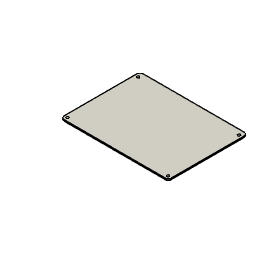
Under Table Mainboard Case - Lid (Autodesk Fusion 360 design; units mm, degrees)
Autodesk Fusion 360 part; units mm, degrees
sketch "Sketch1" plane through (0, 0, 63) normal (0, 0, 1) x (-1, 0, 0)
  circle A0 centre (89, -61) radius 1.925
  circle A1 centre (89, 64) radius 1.925
  circle A2 centre (-89, -61) radius 1.925
  circle A3 centre (-89, 64) radius 1.925
  line L0 (-89, -68.4) -> (-85, -68.4)
  line L1 (-85, -68.4) -> (-85, -67)
  line L2 (-85, -67) -> (-74, -67)
  line L3 (-74, -67) -> (-74, -64)
  line L4 (-74, -64) -> (-83, -64)
  arc A4 (-86, -61) -> (-83, -64) centre (-83, -61) ccw
  arc A5 (-86, -61) -> (-89, -58) centre (-89, -61) ccw
  arc A6 (-92, -55) -> (-89, -58) centre (-89, -55) ccw
  line L5 (-92, -55) -> (-92, 58)
  arc A7 (-89, 61) -> (-92, 58) centre (-89, 58) ccw
  arc A8 (-89, 61) -> (-86, 64) centre (-89, 64) ccw
  arc A9 (-83, 67) -> (-86, 64) centre (-83, 64) ccw
  line L6 (-83, 67) -> (83, 67)
  arc A10 (86, 64) -> (83, 67) centre (83, 64) ccw
  arc A11 (86, 64) -> (89, 61) centre (89, 64) ccw
  arc A12 (92, 58) -> (89, 61) centre (89, 58) ccw
  line L7 (92, 58) -> (92, -55)
  arc A13 (89, -58) -> (92, -55) centre (89, -55) ccw
  arc A14 (89, -58) -> (86, -61) centre (89, -61) ccw
  arc A15 (83, -64) -> (86, -61) centre (83, -61) ccw
  line L8 (83, -64) -> (74, -64)
  line L9 (74, -64) -> (74, -67)
  line L10 (74, -67) -> (85, -67)
  line L11 (85, -67) -> (85, -68.4)
  line L12 (85, -68.4) -> (89, -68.4)
  arc A16 (89, -68.4) -> (93.4, -64) centre (89, -64) ccw
  line L13 (93.4, -64) -> (93.4, 64)
  arc A17 (93.4, 64) -> (89, 68.4) centre (89, 64) ccw
  line L14 (89, 68.4) -> (-89, 68.4)
  arc A18 (-89, 68.4) -> (-93.4, 64) centre (-89, 64) ccw
  line L15 (-93.4, 64) -> (-93.4, -64)
  arc A19 (-93.4, -64) -> (-89, -68.4) centre (-89, -64) ccw
  line L16 (89, -68.4) -> (85, -68.4)
  arc A20 (89, -68.4) -> (93.4, -64) centre (89, -64) ccw
  line L17 (93.4, 64) -> (93.4, -64)
  arc A21 (93.4, 64) -> (89, 68.4) centre (89, 64) ccw
  line L18 (-89, 68.4) -> (89, 68.4)
  arc A22 (-89, 68.4) -> (-93.4, 64) centre (-89, 64) ccw
  line L19 (-93.4, -64) -> (-93.4, 64)
  arc A23 (-93.4, -64) -> (-89, -68.4) centre (-89, -64) ccw
  line L20 (-85, -68.4) -> (-89, -68.4)
  line L21 (84.75, -68.4) -> (-84.75, -68.4)
  circle A24 centre (-89, -61) radius 1.925
  circle A25 centre (89, -61) radius 1.925
  circle A26 centre (89, 64) radius 1.925
  circle A27 centre (-89, 64) radius 1.925
  line L22 (89, -68.1) -> (85, -68.1)
  arc A28 (89, -68.1) -> (93.1, -64) centre (89, -64) ccw
  line L23 (93.1, -64) -> (93.1, 64)
  arc A29 (93.1, 64) -> (89, 68.1) centre (89, 64) ccw
  line L24 (89, 68.1) -> (-89, 68.1)
  arc A30 (-89, 68.1) -> (-93.1, 64) centre (-89, 64) ccw
  line L25 (-93.1, 64) -> (-93.1, -64)
  arc A31 (-93.1, -64) -> (-89, -68.1) centre (-89, -64) ccw
  line L26 (-89, -68.1) -> (-85, -68.1)
  line L27 (85, -68.1) -> (-85, -68.1)
  dimension "d106" = -0.3
  constraint perpendicular L1 L27
extrude "Extrude1" add sketch "Sketch1" along normal blind 2.2 contours L1 L2 L3 L4 A4 A5 A6 L5 A7 A8 A9 L6 A10 A11 A12 L7 A13 A14 A15 L8 L9 L10 L11 L22 A28 L23 A29 L24 A30 L25 A31 L26 | L1 L2 L3 L4 A4 A5 A6 L5 A7 A8 A9 L6 A10 A11 A12 L7 A13 A14 A15 L8 L9 L10 L11 L27
sketch "Sketch2" plane through (0, 0, 65.2) normal (0, 0, 1) x (-1, 0, 0)
  circle A0 centre (89, -61) radius 1.925
  circle A1 centre (89, 64) radius 1.925
  circle A2 centre (-89, 64) radius 1.925
  circle A3 centre (-89, -61) radius 1.925
  arc A4 (89, -68.1) -> (93.1, -64) centre (89, -64) ccw
  line L0 (93.1, -64) -> (93.1, 64)
  arc A5 (93.1, 64) -> (89, 68.1) centre (89, 64) ccw
  line L1 (89, 68.1) -> (-89, 68.1)
  arc A6 (-89, 68.1) -> (-93.1, 64) centre (-89, 64) ccw
  line L2 (-93.1, 64) -> (-93.1, -64)
  arc A7 (-93.1, -64) -> (-89, -68.1) centre (-89, -64) ccw
  line L3 (-89, -68.1) -> (89, -68.1)
  line L4 (-95, 64) -> (-95, -64)
  arc A8 (-95, -64) -> (-89, -70) centre (-89, -64) ccw
  line L5 (-89, -70) -> (-85, -70)
  line L6 (-84.75, -70) -> (84.75, -70)
  line L7 (85, -70) -> (89, -70)
  arc A9 (89, -70) -> (95, -64) centre (89, -64) ccw
  line L8 (95, -64) -> (95, 64)
  arc A10 (95, 64) -> (89, 70) centre (89, 64) ccw
  line L9 (89, 70) -> (-89, 70)
  arc A11 (-89, 70) -> (-95, 64) centre (-89, 64) ccw
  line L10 (-84.75, -70) -> (-85, -70)
  line L11 (85, -70) -> (84.75, -70)
  constraint coincident L6.start L10.start
  constraint coincident L5.end L10.end
  constraint coincident L7.start L11.start
  constraint coincident L6.end L11.end
extrude "Extrude2" add sketch "Sketch2" along normal blind 2 contours A4 L0 A5 L1 A6 L2 A7 L3 | L4 A8 L5 L6 L7 A9 L8 A10 L9 A11 L10 L11
sketch "Sketch3" plane through (0, 0, 67.2) normal (0, 0, 1) x (-1, 0, 0)
  circle A0 centre (-89, -61) radius 1.925
  circle A1 centre (89, -61) radius 1.925
  circle A2 centre (89, 64) radius 1.925
  circle A3 centre (-89, 64) radius 1.925
  arc A4 (89, -70) -> (95, -64) centre (89, -64) ccw
  line L0 (95, -64) -> (95, 64)
  arc A5 (95, 64) -> (89, 70) centre (89, 64) ccw
  line L1 (89, 70) -> (-89, 70)
  arc A6 (-89, 70) -> (-95, 64) centre (-89, 64) ccw
  line L2 (-95, 64) -> (-95, -64)
  arc A7 (-95, -64) -> (-89, -70) centre (-89, -64) ccw
  line L3 (-89, -70) -> (89, -70)
  circle A8 centre (89, -61) radius 2.25
  circle A9 centre (-89, -61) radius 2.25
  circle A10 centre (-89, 64) radius 2.25
  circle A11 centre (89, 64) radius 2.25
  dimension "d111" = 4.5
  dimension "d112" = 4.5
  dimension "d113" = 4.5
  dimension "d114" = 4.5
  constraint concentric A1 A8
  constraint concentric A0 A9
  constraint concentric A3 A10
  constraint concentric A2 A11
  measures "d111" diameter of A8
  measures "d112" diameter of A9
  measures "d113" diameter of A10
  measures "d114" diameter of A11
extrude "Extrude3" cut sketch "Sketch3" against normal blind 4.2 contours A8 | A9 | A10 | A11
